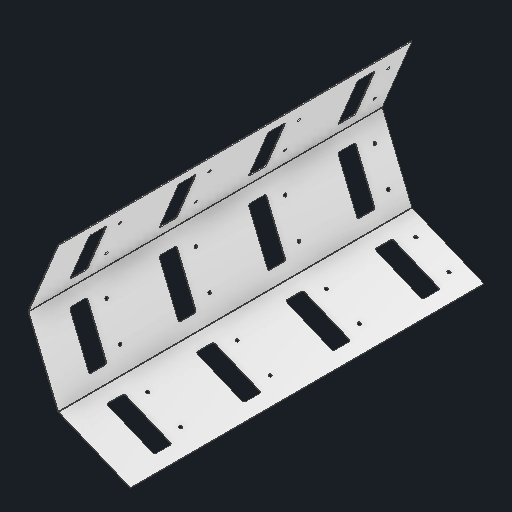
# Autodesk Inventor part: DMF 01 13 Барабан Лист лев брт №2 v2.1
Saved by Autodesk Inventor 2026.2 (Build 302298010, 298A)
## iProperties
Created: 2024-04-28
Part Number: DMF 01 13 Барабан Лист лев брт №2 v2.1
Material: Stainless Steel AISI 304
Document SubType Name: Sheet Metal
Designer: pokla
Stock Number: Барабан_Лист_Левый_Борт
Density: 8 g/cm^3
Flat Pattern Width: 65.4696 cm
Flat Pattern Length: 98.85 cm
Flat Pattern Area: 6471.67 cm^2
Sheet Metal Rule: Default
Sheet Metal Width: 654,696 mm
Sheet Metal Length: 988,500 mm
Sheet Metal Area: 647167,036 mm^2
Appearance: Chrome - Satin
Author: pokla
Autodesk Inventor part; units mm, degrees
note: some values were not read from the file. Chosen so that the rebuilt part matches the saved one: flange form of "Plate6"; pattern direction of "Circular Pattern3".
ref_plane "YZ Plane" through (0, 0, 0) normal (1, 0, 0) x (0, 1, 0)
ref_plane "XZ Plane" through (0, 0, 0) normal (0, 1, 0) x (-1, 0, 0)
ref_plane "XY Plane" through (0, 0, 0) normal (0, 0, 1) x (1, 0, 0)
sketch "Sketch2" plane through (0, 0, 0) normal (0, 0, 1) x (1, 0, 0)
  line L0 (0, 286.8339) -> (202.8222, 202.8222) construction
  line L1 (202.8222, 202.8222) -> (286.8339, 0) construction
  line L2 (286.8339, 0) -> (202.8222, -202.8222) construction
  line L3 (202.8222, -202.8222) -> (0, -286.8339) construction
  line L4 (0, -286.8339) -> (-202.8222, -202.8222) construction
  line L5 (-202.8222, -202.8222) -> (-286.8339, 0) construction
  line L6 (-286.8339, 0) -> (-202.8222, 202.8222) construction
  line L7 (-202.8222, 202.8222) -> (0, 286.8339) construction
  line L8 (-286.1999, -1.5307) -> (-203.4563, -201.2915)
  line L9 (-201.2915, -203.4563) -> (-0.8315, -286.4895)
  arc A0 (-286.1999, 1.5307) -> (-286.1999, -1.5307) centre (-282.5044, 0) ccw
  arc A1 (-203.4563, -201.2915) -> (-201.2915, -203.4563) centre (-199.7608, -199.7608) ccw
  line L10 (-286.1999, 1.5307) -> (-203.1666, 201.9907)
  point P0 (0, 0)
  point P1 (0, 0)
  dimension "d58" = 4
  dimension "d59" = 4
  dimension "d70" = 0.9
  dimension "d72" = 0.9
  dimension "d74" = 530
  measures "d58" radius of A0
  measures "d59" radius of A1
  measures "d70" distance of L3.end L9.end
  measures "d72" distance of L6.end L10.end
  measures "d74" distance between parallel lines of L1 L8
contour flange "Contour Flange3" sketch "Sketch2" thickness 2 bend radius 2 width 988.5 along (0, 0, -1) mid plane no both sides no wall seen from (-101.0615, -244.9729, 0) lies toward (0.3826834, 0.9238795, 0) curves L9 A1 L8 A0 L10
bend "Bend6"
corner "Corner6"
sketch "Sketch15" plane through (-286.1999, -1.5307, -988.5) normal (-0.9238795, -0.3826834, 0) x (0, 0, 1)
  line L0 (838.5, -35.6097) -> (888.5, -35.6097)
  line L1 (888.5, -35.6097) -> (888.5, -180.6097)
  line L2 (888.5, -180.6097) -> (838.5, -180.6097)
  line L3 (838.5, -180.6097) -> (838.5, -35.6097)
  circle A0 centre (793.5, -58.1097) radius 4.5
  circle A1 centre (793.5, -158.1097) radius 4.5
  line L4 (888.5, -108.1097) -> (838.5, -108.1097) construction
  line L5 (0, -216.2195) -> (0, 0) projected
  line L6 (988.5, -216.2195) -> (988.5, 0) projected
  point P0 (0, -108.1097)
  dimension "d192" = 9
  dimension "d193" = 145
  dimension "d194" = 50
  dimension "d195" = 45
  dimension "d196" = 100
  dimension "d207" = 100
  constraints: 10 end point, 3 midpoint, 2 centre point, 2 parallel, 1 horizontal, 1 horizontal alignment, 1 perpendicular, 1 other
  measures "d192" diameter of A0
  measures "d193" distance of L2.end L0.start
  measures "d194" distance of L0.start L0.end
  measures "d195" distance from line of A0.centre L3
  measures "d196" distance of A1.centre A0.centre
  measures "d207" distance between parallel lines of L6 L1
extrude "Cut1" cut sketch "Sketch15" against normal through all
fillet "Fillet2" radius 5 4 edges at (-216.1596, -168.0097, -150) (-216.1596, -168.0097, -100) (-271.6487, -34.0472, -100) (-271.6487, -34.0472, -150)
pattern_linear "Rectangular Pattern3" count 4 spacing 250 along (0, 0, -1) of "Cut1", "Fillet2"
pattern_circular "Circular Pattern3" count 3 over 90 about axis through (0, 0, -10) along (0, 0, 1) of "Cut1", "Rectangular Pattern3", "Fillet2" both ways yes
equation "\"d58\" = BendRadius + Thickness"
equation "\"d59\" = BendRadius + Thickness"
equation "\"d74\" = Барабан_размер_по_плоскостям"
equation "\"d75\" = Thickness"
equation "\"d76\" = BendReliefWidth"
equation "\"d77\" = BendReliefDepth"
equation "\"d78\" = MinimumRemnant"
equation "\"d79\" = TransitionRadius"
equation "\"d81\" = BendRadius"
equation "\"d83\" = CornerReliefSize"
equation "\"d84\" = GapSize"
equation "\"d85\" = JacobiRadiusSize"
equation "\"BendRadius\" = Thickness"
equation "\"BendReliefWidth\" = Thickness"
equation "\"BendReliefDepth\" = 0.5 * Thickness"
equation "\"CornerReliefSize\" = 4 * Thickness"
equation "\"MinimumRemnant\" = 2 * Thickness"
equation "\"TransitionRadius\" = BendRadius"
equation "\"JacobiRadiusSize\" = BendRadius"
equation "\"GapSize\" = Thickness"
equation "\"Барабан_Середина_листа\" = 206.27835"
equation "\"Thickness\" = 2"
equation "\"Барабан_размер_по_плоскостям\" = 530"
body "Solid3"
